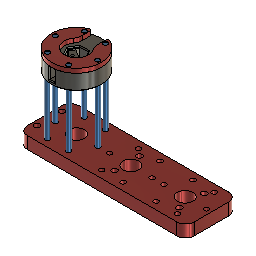
CNC6040ToolChanger (Autodesk Fusion 360 design; units mm, degrees)
Autodesk Fusion 360 part; units mm, degrees
note: some values were not read from the file. Chosen so that the rebuilt part matches the saved one: which face or edge a step refers to.
box "Grundkörper Quader1" add length 60 width 60 height 10 placed x (0, 1, 0) y (-1, 0, 0) z (0, 0, 1) at (60, 0, 0) makes body 1
cylinder "Grundkörper Zylinder3" add diameter 5 height 100.17 placed x (1, 0, 0) y (0, 1, 0) z (0, 0, 1) at (0, 0, 10) separate body makes body 2
move_body "Verschieben2" bodies 2 to x (1, 0, 0) y (0, 1, 0) z (0, 0, 1) at (5.3, 30, -10)
ref_plane "Arbeitsebene1" through (30, 30, 5) normal (0, 1, 0) x (0, 0, -1)
ref_plane "Arbeitsebene2" through (30, 30, 5) normal (1, 0, 0) x (0, 0, -1)
pattern_circular "C-Anordnung1" count 6 over 360 about axis through (30, 30, -0.68) along (0, 0, 1) of bodies 2 makes body 3 at (19.1094, 10.639, 66.78) makes body 4 at (41.3218, 10.8879, 66.78) makes body 5 at (52.2124, 30.2489, 66.78) makes body 6 at (40.8906, 49.361, 66.78) makes body 7 at (18.6782, 49.1121, 66.78)
cylinder "Grundkörper Zylinder4" add diameter 58 height 18 placed x (1, 0, 0) y (0, 1, 0) z (0, 0, 1) at (0, 0, 10) separate body makes body 8
move_body "Verschieben3" bodies 8 to x (1, 0, 0) y (0, 1, 0) z (0, 0, 1) at (30, 30, 67.61)
move_face "Flächen versetzen10" offset 7 1 faces at (0, 40, 3.3333) on bodies 1
move_face "Flächen versetzen11" offset 126.44 1 faces at (60, 40, 3.3333) on bodies 1
shell "Schale1" thickness 9.5 removed faces 1 at (20.8612, 22.9565, 95.61) on bodies 8
move_face "Flächen versetzen8" offset 14.59 1 faces at (49.4031, 28.0584, 89.9433) on bodies 8
cylinder "Grundkörper Zylinder5" add diameter 5.45 height -124.25 placed x (1, 0, 0) y (0, 1, 0) z (0, 0, 1) at (5, 30, 100.17) separate body makes body 9
move_body "Verschieben10" bodies 9 to x (1, 0, 0) y (0, 1, 0) z (0, 0, 1) at (0.3, 0, 0)
move_body "Verschieben28" bodies 9 to x (1, 0, 0) y (0, 1, 0) z (0, 0, 1) at (0, 0, -0.52)
pattern_circular "C-Anordnung2" count 6 over 360 about axis through (30, 30, -0.68) along (0, 0, 1) of bodies 9 makes body 10 at (19.2407, 10.8217, 58.2333) makes body 11 at (41.2292, 11.093, 58.2333) makes body 12 at (51.9885, 30.2713, 58.2333) makes body 13 at (40.7593, 49.1783, 58.2333) makes body 14 at (15.139, 52.4493, 16.8167)
cylinder "Grundkörper Zylinder12" add diameter 58 height 5 placed x (1, 0, 0) y (0, 1, 0) z (0, 0, 1) at (30, 30, 95.61) separate body makes body 15
cylinder "Grundkörper Zylinder16" add diameter 61 height 6.3 placed x (1, 0, 0) y (0, 1, 0) z (0, 0, 1) at (30, 30, 10) separate body makes body 16
move_body "Verschieben26" bodies 16 to x (1, 0, 0) y (0, 1, 0) z (0, 0, 1) at (0, 0, 47.5)
hole "Bohrung10" at (30, 30, 63.8) direction (0, 0, -1) diameter 34.12 depth 20 tip angle 118 bodies 16
combine "Kombinieren7" operation cut target body 16 tool bodies 10 11 12 13 14 9 keep tools
combine "Kombinieren1" operation cut target body 15 tool bodies 9 14 13 12 11 10 keep tools
move_body "Verschieben64" bodies 14 13 12 11 10 9 to x (1, 0, 0) y (0, 1, 0) z (0, 0, 1) at (0, 0, 3.93)
combine "Kombinieren22" operation cut target body 15 tool bodies 10 11 12 13 14 9 keep tools
copy_body "Körper kopieren/einfügen39" bodies 11 9 14 12 13 10 makes body 17 makes body 18 makes body 19 makes body 20 makes body 21 makes body 22
move_face "Flächen versetzen15" offset 0.2 1 faces at (19.2407, 10.8217, 62.1633) on bodies 22
move_face "Flächen versetzen16" offset 0.2 1 faces at (8.0115, 29.7287, 62.1633) on bodies 18
move_face "Flächen versetzen17" offset 0.2 1 faces at (15.139, 52.4493, 20.7467) on bodies 19
move_face "Flächen versetzen18" offset 0.2 1 faces at (40.7593, 49.1783, 62.1633) on bodies 21
move_face "Flächen versetzen19" offset 0.2 1 faces at (51.9885, 30.2713, 62.1633) on bodies 20
move_face "Flächen versetzen20" offset 0.2 1 faces at (41.2292, 11.093, 62.1633) on bodies 17
combine "Kombinieren34" operation cut target body 8 tool bodies 22 18 19 21 20 17
chamfer "Fase4" distance 1 angle 45 1 edges at (2.9625, 40.4868, 77.61) on bodies 8
sketch "Skizze64" plane through (0, 0, 95.41) normal (0, 0, 1) x (-1, 0, 0)
  line L0 (-40.0459, -29.9999) -> (-35.023, -38.7)
  line L1 (-35.023, -38.7) -> (-24.9771, -38.7)
  line L2 (-24.9771, -38.7) -> (-19.9541, -30.0001)
  line L3 (-19.9541, -30.0001) -> (-24.977, -21.3)
  line L4 (-24.977, -21.3) -> (-35.0229, -21.3)
  line L5 (-35.0229, -21.3) -> (-40.0459, -29.9999)
  circle A0 centre (-30, -30) radius 14
  point P0 (-30, -30)
  dimension "d142" = 8.7
  constraint coincident P0 A0.centre
  measures "d142" distance of P0 L5
extrude "Extrusion2" add sketch "Skizze64" along normal blind 28 separate body contours L0 L1 L2 L3 L4 L5 makes body 23
move_body "Verschieben22" bodies 23 to x (1, 0, 0) y (0, 1, 0) z (0, 0, 1) at (0, 0, -25.99)
move_face "Flächen versetzen21" offset 0.2 6 faces at (21.6284, 27.1001, 78.7533) (28.3256, 21.3, 78.7533) (36.6972, 24.2, 78.7533) (38.3716, 32.8999, 78.7533) (31.6744, 38.7, 78.7533) (23.3028, 35.8, 78.7533) on bodies 23
combine "Kombinieren17" operation cut target body 8 tool bodies 23
chamfer "Fase13" distance 1 angle 45 6 edges at (22.2924, 34.4501, 95.61) (30.0001, 38.9, 95.61) (37.7077, 34.4499, 95.61) (37.7076, 25.5499, 95.61) (29.9999, 21.1, 95.61) (22.2923, 25.5501, 95.61) on bodies 8
hole "Bohrung8" at (30, 30, 100.61) direction (0, 0, -1) diameter 27.96 depth 72.03 tip angle 118 bodies 15
chamfer "Fase15" distance 1 angle 45 1 edges at (1.564, 41.0293, 57.5) on bodies 16
cylinder "Grundkörper Zylinder17" add diameter 2.9 height 20.71 placed x (0, 0, -1) y (0, 1, 0) z (1, 0, 0) at (0, 29.93, 59.9) separate body makes body 24
move_body "Verschieben27" bodies 24 to x (1, 0, 0) y (0, 1, 0) z (0, 0, 1) at (6.16, 0, 0.76)
pattern_circular "C-Anordnung10" count 6 over 360 about axis through (30, 30, -0.68) along (0, 0, 1) of bodies 24 makes body 25 at (20.3556, 16.0114, 60.9118) makes body 26 at (37.283, 14.648, 60.4797) makes body 27 at (46.9367, 28.642, 60.4082) makes body 28 at (34.831, 38.7963, 59.2172) makes body 29 at (20.2251, 43.9132, 60.4797)
combine "Kombinieren18" operation cut target body 16 tool bodies 24 25 26 27 28 29
chamfer "Fase14" distance 1.69 angle 45 6 edges at (12.9959, 31.38, 60.66) (22.6931, 45.416, 60.66) (39.6972, 44.036, 60.66) (47.0041, 28.62, 60.66) (37.3069, 14.584, 60.66) (20.3028, 15.964, 60.66) on bodies 16
box "Grundkörper Quader4" add length 6.42 width 14 height -9.01 placed x (0, 1, 0) y (-1, 0, 0) z (0, 0, 1) at (37.37, 5.48, 63.8) separate body makes body 30
box "Grundkörper Quader5" add length 3.28 width 13.98 height 3.51 placed x (0, 1, 0) y (1, 0, 0) z (0, 0, -1) at (23.36, 6.99, 54.79) bodies 30
copy_body "Körper kopieren/einfügen10" bodies 30 makes body 31
move_body "Verschieben29" bodies 31 to x (1, 0, 0) y (0, 1, 0) z (0, 0, 1) at (0, 0, 3.97)
move_face "Flächen versetzen9" offset 7.19 1 faces at (32.68, 8.0833, 55.25) on bodies 31
combine "Kombinieren23" operation cut target body 16 tool bodies 31
move_body "Verschieben30" bodies 30 to x (1, 0, 0) y (0, 1, 0) z (0, 0, 1) at (0, 0, 3.38)
box "Grundkörper Quader6" add length 4.25 width 0.92 height 0.71 placed x (0, -1, 0) y (1, 0, 0) z (0, 0, 1) at (26.41, 10.96, 67.18) bodies 30
box "Grundkörper Quader7" add length 12.64 width 4.61 height -0.13 placed x (0, 0, 1) y (0, 1, 0) z (-1, 0, 0) at (23.37, 6.57, 68.04) separate body makes body 32
move_body "Verschieben31" bodies 32 to x (0.258819, 0, -0.965926) y (0, 1, 0) z (0.965926, 0, 0.258819) at (-47.6024, 0, 72.7683)
combine "Kombinieren24" operation add target body 32 tool bodies 30 makes body 33 at (28.0367, 5.48, 61.1733)
cylinder "Grundkörper Zylinder18" add diameter 61 height 31.81 placed x (1, 0, 0) y (0, 1, 0) z (0, 0, 1) at (30, 30, 63.8) separate body makes body 34
hole "Bohrung11" at (30, 30, 95.61) direction (0, 0, -1) diameter 59.4 depth 58.86 tip angle 118 bodies 34
combine "Kombinieren21" operation add target body 16 tool bodies 34
box "Grundkörper Quader8" add length 148.44 width 696.14 height -33.22 placed x (0, -1, 0) y (1, 0, 0) z (0, 0, 1) at (0, 0, 0) separate body makes body 35
cylinder "Grundkörper Zylinder23" add diameter 2.5 height 1.91 placed x (0, 1, 0) y (1, 0, 0) z (0, 0, -1) at (35.486, 8.5789, 77.61) separate body makes body 36
cylinder "Grundkörper Zylinder24" add diameter 4.5 height 0.98 placed x (0, 1, 0) y (1, 0, 0) z (0, 0, -1) at (35.486, 8.5789, 75.7) bodies 36
cylinder "Grundkörper Zylinder19" add diameter 6.3 height 18.31 placed x (1, 0, 0) y (0, 1, 0) z (0, 0, 1) at (6.09, -11.75, 0) separate body makes body 37
cylinder "Grundkörper Zylinder21" add diameter 11 height 5.49 placed x (1, 0, 0) y (0, 1, 0) z (0, 0, 1) at (6.09, -11.75, 18.31) bodies 37
copy_body "Körper kopieren/einfügen11" bodies 37 makes body 38
move_body "Verschieben32" bodies 38 to x (1, 0, 0) y (0, 1, 0) z (0, 0, 1) at (45, 0, 0)
copy_body "Körper kopieren/einfügen12" bodies 38 makes body 39
move_body "Verschieben33" bodies 39 to x (1, 0, 0) y (0, 1, 0) z (0, 0, 1) at (45, 0, 0)
copy_body "Körper kopieren/einfügen13" bodies 39 makes body 40
move_body "Verschieben34" bodies 40 to x (1, 0, 0) y (0, 1, 0) z (0, 0, 1) at (30, 0, 0)
copy_body "Körper kopieren/einfügen14" bodies 40 makes body 41
move_body "Verschieben35" bodies 41 to x (1, 0, 0) y (0, 1, 0) z (0, 0, 1) at (45, 0, 0)
copy_body "Körper kopieren/einfügen15" bodies 41 makes body 42
move_body "Verschieben36" bodies 42 to x (1, 0, 0) y (0, 1, 0) z (0, 0, 1) at (45, 0, 0)
copy_body "Körper kopieren/einfügen16" bodies 42 makes body 43
move_body "Verschieben37" bodies 43 to x (1, 0, 0) y (0, 1, 0) z (0, 0, 1) at (30, 0, 0)
copy_body "Körper kopieren/einfügen17" bodies 43 makes body 44
move_body "Verschieben38" bodies 44 to x (1, 0, 0) y (0, 1, 0) z (0, 0, 1) at (45, 0, 0)
copy_body "Körper kopieren/einfügen18" bodies 44 makes body 45
move_body "Verschieben39" bodies 45 to x (1, 0, 0) y (0, 1, 0) z (0, 0, 1) at (45, 0, 0)
copy_body "Körper kopieren/einfügen19" bodies 45 makes body 46
move_body "Verschieben40" bodies 46 to x (1, 0, 0) y (0, 1, 0) z (0, 0, 1) at (30, 0, 0)
copy_body "Körper kopieren/einfügen27" bodies 46 makes body 47
move_body "Verschieben50" bodies 47 to x (1, 0, 0) y (0, 1, 0) z (0, 0, 1) at (45, 0, 0)
copy_body "Körper kopieren/einfügen28" bodies 47 makes body 48
move_body "Verschieben51" bodies 48 to x (1, 0, 0) y (0, 1, 0) z (0, 0, 1) at (45, 0, 0)
combine "Kombinieren25" operation add target body 46 tool bodies 41 40 44 42 43 45 39 38 37 35 47 48
box "Grundkörper Quader15" cut length 29.91 width 18 height -6.71 placed x (0, 1, 0) y (-1, 0, 0) z (0, 0, 1) at (39.01, 39.69, 100.61) bodies 15
fillet "Abrundung13" radius 14 2 edges at (21.01, 40.7061, 98.11) (39.01, 40.6893, 98.11) on bodies 15
fillet "Abrundung14" radius 2 2 edges at (39.01, 57.5648, 98.11) (21.01, 57.5714, 98.11) on bodies 15
copy_body "Körper kopieren/einfügen23" bodies 2 5 3 4 6 7 8 15 16 makes body 49 makes body 50 makes body 51 makes body 52 makes body 53 makes body 54 makes body 55 makes body 56 makes body 57
move_body "Verschieben45" bodies 49 50 51 52 53 54 55 56 57 to x (1, 0, 0) y (0, 1, 0) z (0, 0, 1) at (63, 0, 0)
copy_body "Körper kopieren/einfügen24" bodies 2 5 3 4 6 7 8 15 16 makes body 58 makes body 59 makes body 60 makes body 61 makes body 62 makes body 63 makes body 64 makes body 65 makes body 66
move_body "Verschieben46" bodies 58 59 60 61 62 63 64 65 66 to x (1, 0, 0) y (0, 1, 0) z (0, 0, 1) at (126, 0, 0)
move_body "Verschieben47" bodies 46 to x (1, 0, 0) y (0, 1, 0) z (0, 0, 1) at (-7.48, 27.35, -3.51)
move_face "Flächen versetzen14" offset 4 1 faces at (57.48, 20, 10) on bodies 1
copy_body "Körper kopieren/einfügen25" bodies 66 65 64 63 62 61 60 59 58 57 56 55 54 53 52 51 50 49 32 16 15 8 1 7 6 5 4 3 2 makes body 67 makes body 68 makes body 69 makes body 70 makes body 71 makes body 72 makes body 73 makes body 74 makes body 75 makes body 76 makes body 77 makes body 78 makes body 79 makes body 80 makes body 81 makes body 82 makes body 83 makes body 84 makes body 85 makes body 86 makes body 87 makes body 88 makes body 89 makes body 90 makes body 91 makes body 92 makes body 93 makes body 94 makes body 95
move_body "Verschieben48" bodies 67 68 69 70 71 72 73 74 75 76 77 78 79 80 81 82 83 84 85 86 87 88 89 90 91 92 93 94 95 to x (1, 0, 0) y (0, 1, 0) z (0, 0, 1) at (189, 0, 0)
copy_body "Körper kopieren/einfügen26" bodies 46 makes body 96
move_body "Verschieben49" bodies 96 to x (1, 0, 0) y (0, 1, 0) z (0, 0, 1) at (0, 28.9, 0)
combine "Kombinieren26" operation add target body 46 tool bodies 96
copy_body "Körper kopieren/einfügen29" bodies 75 74 73 71 72 69 70 68 67 makes body 97 makes body 98 makes body 99 makes body 100 makes body 101 makes body 102 makes body 103 makes body 104 makes body 105
move_body "Verschieben52" bodies 97 98 99 100 101 102 103 104 105 to x (1, 0, 0) y (0, 1, 0) z (0, 0, 1) at (63, 0, 0)
move_face "Flächen versetzen12" offset -6.52 1 faces at (182, 40, 4.6667) on bodies 89
move_face "Flächen versetzen13" offset 63.07 1 faces at (375.44, 40, 4.6667) on bodies 89
fillet "Abrundung11" radius 10 8 edges at (-7, 0, 5) (-7, 60, 5) (186.44, 0, 5) (186.44, 60, 5) (188.52, 60, 7) (188.52, 0, 7) (438.51, 0, 7) (438.51, 60, 7) on bodies 1 89
box "Grundkörper Quader9" cut length 100.97 width 15.93 height 31.52 placed x (0, 1, 0) y (-1, 0, 0) z (0, 0, 1) at (49.94, -19.79, -3.51) bodies 46
box "Grundkörper Quader10" cut length 96.45 width 17.32 height 25.46 placed x (0, 1, 0) y (-1, 0, 0) z (0, 0, 1) at (214.86, -8.85, -3.51) bodies 46
box "Grundkörper Quader11" cut length 98.18 width 27.62 height 30.74 placed x (0, 1, 0) y (-1, 0, 0) z (0, 0, 1) at (371.77, -23.83, -3.51) bodies 46
box "Grundkörper Quader12" cut length 135.28 width 16.09 height 33.65 placed x (0, 1, 0) y (-1, 0, 0) z (0, 0, 1) at (128.73, -29.44, -3.51) bodies 46
box "Grundkörper Quader13" cut length 128.05 width 15.39 height 26.28 placed x (0, 1, 0) y (-1, 0, 0) z (0, 0, 1) at (293.14, -11.78, -3.51) bodies 46
combine "Kombinieren27" operation cut target body 1 tool bodies 46 keep tools
combine "Kombinieren28" operation cut target body 89 tool bodies 46 keep tools
cylinder "Grundkörper Zylinder22" add diameter 18 height -26.72 placed x (1, 0, 0) y (0, 1, 0) z (0, 0, 1) at (30, 30, 10) separate body makes body 106
move_body "Verschieben61" bodies 106 to x (1, 0, 0) y (0, 1, 0) z (0, 0, 1) at (0, 0, 9.29)
copy_body "Körper kopieren/einfügen30" bodies 106 makes body 107
move_body "Verschieben53" bodies 107 to x (1, 0, 0) y (0, 1, 0) z (0, 0, 1) at (63, 0, 0)
copy_body "Körper kopieren/einfügen31" bodies 107 makes body 108
move_body "Verschieben54" bodies 108 to x (1, 0, 0) y (0, 1, 0) z (0, 0, 1) at (63, 0, 0)
copy_body "Körper kopieren/einfügen32" bodies 108 makes body 109
move_body "Verschieben55" bodies 109 to x (1, 0, 0) y (0, 1, 0) z (0, 0, 1) at (63, 0, 0)
copy_body "Körper kopieren/einfügen33" bodies 109 makes body 110
move_body "Verschieben56" bodies 110 to x (1, 0, 0) y (0, 1, 0) z (0, 0, 1) at (63, 0, 0)
copy_body "Körper kopieren/einfügen34" bodies 110 makes body 111
move_body "Verschieben57" bodies 111 to x (1, 0, 0) y (0, 1, 0) z (0, 0, 1) at (63, 0, 0)
copy_body "Körper kopieren/einfügen35" bodies 111 makes body 112
move_body "Verschieben58" bodies 112 to x (1, 0, 0) y (0, 1, 0) z (0, 0, 1) at (63, 0, 0)
combine "Kombinieren29" operation cut target body 1 tool bodies 106 107 108
combine "Kombinieren30" operation cut target body 89 tool bodies 109 110 111 112
copy_body "Körper kopieren/einfügen36" bodies 10 14 13 12 11 9 makes body 113 makes body 114 makes body 115 makes body 116 makes body 117 makes body 118
move_body "Verschieben59" bodies 113 114 115 116 117 118 to x (1, 0, 0) y (0, 1, 0) z (0, 0, 1) at (63, 0, 0)
copy_body "Körper kopieren/einfügen37" bodies 113 116 115 114 117 118 makes body 119 makes body 120 makes body 121 makes body 122 makes body 123 makes body 124
move_body "Verschieben60" bodies 119 120 121 122 123 124 to x (1, 0, 0) y (0, 1, 0) z (0, 0, 1) at (63, 0, 0)
combine "Kombinieren31" operation cut target body 1 tool bodies 11 10 9 14 13 12 118 114 113 115 116 117 124 119 122 123 120 121 keep tools
move_body "Verschieben62" bodies 121 124 122 123 119 120 114 113 115 116 117 12 118 13 14 9 10 11 to x (1, 0, 0) y (0, 1, 0) z (0, 0, 1) at (189, 0, 0)
copy_body "Körper kopieren/einfügen38" bodies 121 123 120 122 119 124 makes body 125 makes body 126 makes body 127 makes body 128 makes body 129 makes body 130
move_body "Verschieben63" bodies 125 126 127 128 129 130 to x (1, 0, 0) y (0, 1, 0) z (0, 0, 1) at (63, 0, 0)
combine "Kombinieren32" operation cut target body 89 tool bodies 11 125 127 126 124 10 122 123 119 120 121 114 113 115 116 9 14 117 12 118 13 128 129 130
cylinder "Grundkörper Zylinder25" add diameter 10 height 9 placed x (1, 0, 0) y (0, 1, 0) z (0, 0, 1) at (20.83, -27.86, -3.51) separate body makes body 131
hole "Bohrung16" at (20.83, -27.86, 5.49) direction (0, 0, -1) diameter 5.6 depth 19.97 tip angle 118 bodies 46 131
move_face "Flächen versetzen23" offset 0.2 6 faces at (31.7127, 21.1, 88.9433) (23.1487, 24.0667, 83.2767) (21.436, 32.9667, 83.2767) (31.7129, 38.9, 88.9433) (36.8513, 35.9333, 88.9433) (36.8512, 24.0666, 83.2767) on bodies 8
box "Grundkörper Quader16" add length 13 width 6 height -39.1 placed x (0, 0, 1) y (1, -0.000007, 0) z (0.000007, 1, 0) at (29.1384, 21.1, 77.61) separate body makes body 132
move_body "Verschieben65" bodies 132 to x (1, 0, 0) y (0, 1, 0) z (0, 0, 1) at (-2.11, 4.7, 3.87)
combine "Kombinieren35" operation cut target body 8 tool bodies 132
fillet "Abrundung15" radius 1 4 edges at (27.0282, 1.1527, 87.98) (30.0283, 1, 94.48) (33.0282, 1.1585, 87.98) (30.0283, 1, 81.48) on bodies 8
hole "Bohrung17" at (29.9981, 18.1, 77.61) direction (0, 0, 1) diameter 2.7 depth 6.38 tip angle 118 bodies 8
move_face "Flächen versetzen22" offset 0.15 6 faces at (51.7895, 30.2912, 89.61) (8.2105, 29.7088, 89.61) (19.3575, 10.9841, 89.61) (18.853, 48.7247, 89.61) (41.8421, 5.7286, 83.61) (40.6425, 49.0159, 89.61) on bodies 8
move_face "Flächen versetzen24" offset 0.1 6 faces at (8.0115, 29.7287, 98.9433) (15.0893, 52.3228, 97.2767) (40.7593, 49.1783, 98.9433) (51.9885, 30.2713, 98.9433) (41.2292, 11.093, 98.9433) (19.2407, 10.8217, 98.9433) on bodies 15
box "Grundkörper Quader17" add length 9.15 width 9.15 height 38.41 placed x (0, 0, -1) y (-0.500006, -0.866022, 0) z (-0.866022, 0.500006, 0) at (39.824, 29.6156, 94.61) separate body makes body 133
move_body "Verschieben70" bodies 133 to x (1, 0, 0) y (0, 1, 0) z (0, 0, 1) at (8.92, -5.1501, -1)
combine "Kombinieren36" operation cut target body 8 tool bodies 133
hole "Bohrung18" at (40.9954, 23.6446, 77.61) direction (0, 0, 1) diameter 2.7 depth 11.04 tip angle 118 bodies 8
hole "Bohrung19" at (19.0101, 36.3649, 77.61) direction (0, 0, 1) diameter 2.7 depth 11.04 tip angle 118 bodies 8
hidden bodies 16 32 33 36 46 49 50 51 52 53 54 55 56 57 58 59 60 61 62 63 64 65 66 67 68 69 70 71 72 73 74 75 76 77 78 79 80 81 82 83 84 85 86 87 88 89 90 91 92 93 94 95 97 98 99 100 101 102 103 104 105 131
named bodies: "Grundplatte", "Bolzen (5)", "Bolzen (4)", "Bolzen (3)", "Bolzen (2)", "Kranz", "Bolzen (1)", "Bolzen", "Deckel", "Hex", "Federring", "Bolzen (5) (1)", "Bolzen (2) (1)", "Bolzen (4) (1)", "Bolzen (3) (1)", "Bolzen (1) (1)", "Bolzen (6)", "Kranz (1)", "Deckel (1)", "Federring (1)", "Bolzen (5) (1) (1)", "Bolzen (2) (1) (1)", "Bolzen (4) (1) (1)", "Bolzen (3) (1) (1)", "Bolzen (1) (1) (1)", "Bolzen (6) (1)", "Kranz (1) (1)", "Deckel (1) (1)", "Federring (1) (1)", "Federring (1) (2)", "Deckel (1) (2)", "Kranz (1) (2)", "Bolzen (6) (2)", "Bolzen (1) (1) (2)", "Bolzen (3) (1) (2)", "Bolzen (4) (1) (2)", "Bolzen (2) (1) (2)", "Bolzen (5) (1) (2)", "Federring (2)", "Deckel (2)", "Kranz (2)", "Bolzen (7)", "Bolzen (1) (2)", "Bolzen (2) (2)", "Bolzen (3) (2)", "Bolzen (4) (2)", "Bolzen (5) (2)", "Federring (1) (1) (1)", "Deckel (1) (1) (1)", "Kranz (1) (1) (1)", "Bolzen (6) (1) (1)", "Bolzen (1) (1) (1) (1)", "Bolzen (3) (1) (1) (1)", "Bolzen (4) (1) (1) (1)", "Bolzen (2) (1) (1) (1)", "Bolzen (5) (1) (1) (1)", "Grundplattex4", "Bolzen (5) (1) (1) (1) (1)", "Bolzen (2) (1) (1) (1) (1)", "Bolzen (4) (1) (1) (1) (1)", "Bolzen (1) (1) (1) (1) (1)", "Bolzen (3) (1) (1) (1) (1)", "Kranz (1) (1) (1) (1)", "Bolzen (6) (1) (1) (1)", "Deckel (1) (1) (1) (1)", "Federring (1) (1) (1) (1)", "Stellschraube", "DistanzStück"
